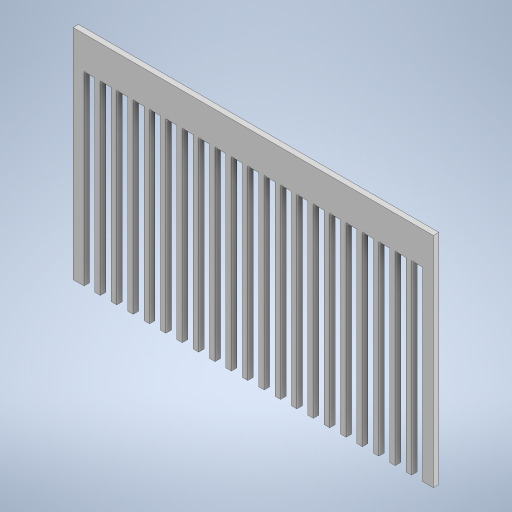
# Autodesk Inventor part: 猫铲
Saved by Autodesk Inventor 2023.1 (Build 271208000, 208)
## iProperties
Created: 2023-07-14
Part Number: 猫铲
Material: 常规
Document SubType Name: Modeling
Designer: Selcon
Density: 1 g/cm^3
Appearance: 默认
Author: Selcon
Autodesk Inventor part; units mm, degrees
ref_plane "YZ Plane" through (0, 0, 0) normal (1, 0, 0) x (0, 1, 0)
ref_plane "XZ Plane" through (0, 0, 0) normal (0, 1, 0) x (-1, 0, 0)
ref_plane "XY Plane" through (0, 0, 0) normal (0, 0, 1) x (1, 0, 0)
sketch "草图1" plane through (0, 0, 0) normal (0, 0, 1) x (1, 0, 0)
  line L0 (-165, 200) -> (165, 200)
  line L1 (165, 200) -> (165, 0)
  line L2 (165, 0) -> (-165, 0)
  line L3 (-165, 0) -> (-165, 200)
  line L4 (0, -40) -> (0, 240) projected
  line L5 (-231, 0) -> (231, 0) projected
  point P0 (0, 0)
  dimension "d0" = 330
  dimension "d1" = 200
  dimension "d2" = 200
  constraints: 8 end point, 2 parallel, 1 horizontal, 1 perpendicular, 1 other
  measures "d0" distance of L0.start L0.end
  measures "d1" distance of L0.end L1.end
  measures "d2" distance between parallel lines of L5 L0
extrude "拉伸1" add sketch "草图1" along normal blind 5
sketch "草图2" plane through (0, 0, 5) normal (0, 0, 1) x (1, 0, 0)
  line L0 (-155, 170) -> (-145, 170)
  line L1 (-145, 170) -> (-145, 0)
  line L2 (-145, 0) -> (-155, 0)
  line L3 (-155, 0) -> (-155, 170)
  line L4 (-165, 200) -> (-165, 0) projected
  line L5 (165, 200) -> (-165, 200) projected
  point P0 (0, 0)
  point P1 (-150, 170)
  dimension "d5" = 10
  dimension "d6" = 10
  dimension "d7" = 30
  constraints: 8 end point, 2 parallel, 1 horizontal, 1 midpoint, 1 perpendicular
  measures "d5" distance between parallel lines of L3 L4
  measures "d6" distance of L1.end L2.end
  measures "d7" distance from line of L5 point (-150, 170)
extrude "拉伸2" cut sketch "草图2" against normal through all
pattern_linear "矩形阵列1" count 21 spacing 15 along (1, 0, 0) of "拉伸2"
